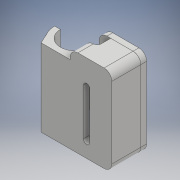
# Autodesk Inventor part: br
Saved by Autodesk Inventor 2018 (Build 220112000, 112)
## iProperties
Created: 2018-02-02
Part Number: br
Material: Generic
Document SubType Name: Modeling
Designer: eroldan
Density: 1 g/cm^3
Appearance: Default
Author: eroldan
Autodesk Inventor part; units mm, degrees
ref_plane "YZ Plane" through (0, 0, 0) normal (1, 0, 0) x (0, 1, 0)
ref_plane "XZ Plane" through (0, 0, 0) normal (0, 1, 0) x (-1, 0, 0)
sketch "Sketch4" plane through (0, 0, 0) normal (0, 0, 1) x (1, 0, 0)
  arc A0 (-8, 0) -> (8, 0) centre (0, 0) ccw
  line L0 (-11, 0) -> (-8, 0)
  line L1 (7.5498, -8) -> (25.5498, -8)
  line L2 (25.5498, -8) -> (25.5498, -11)
  arc A1 (-11, 0) -> (-9.5, -5.5453) centre (0, 0) ccw
  arc A2 (7.5498, -8) -> (11, 0) centre (0, 0) ccw
  line L3 (8, 0) -> (11, 0)
  line L4 (-7.0263, -11) -> (-9.5, -5.5453)
  line L5 (-7.0263, -11) -> (25.5498, -11)
  dimension "d0" = 16
  dimension "d14" = 18
  dimension "d15" = 3
  dimension "d20" = 3
  constraints: 12 end point, 6 point on circle, 4 horizontal, 3 centre point, 1 coincident, 1 perpendicular
  measures "d0" diameter of A0
  measures "d14" distance of L1.start L1.end
  measures "d15" distance of L1.end L2.end
  measures "d20" radial gap between concentric circles of A2 A0
extrude "Extrusion1" add sketch "Sketch4" along normal blind 40
sketch "Sketch5" plane through (7.5498, -8, 0) normal (0, 1, 0) x (1, 0, 0)
  line L0 (0, 0) -> (18, 0) projected
  line L1 (0, 0) -> (0, -40) projected
  line L2 (18, -40) -> (0, -40) projected
  line L3 (18, 0) -> (18, -40) projected
  line L4 (9, -32) -> (9, -8) construction
  line L5 (10.65, -32) -> (10.65, -8)
  line L6 (7.35, -8) -> (7.35, -32)
  arc A0 (7.35, -32) -> (10.65, -32) centre (9, -32) ccw
  arc A1 (10.65, -8) -> (7.35, -8) centre (9, -8) ccw
  point P0 (-7.5498, 0)
  point P1 (9, -20)
  point P2 (18, -20)
  dimension "d5" = 9
  dimension "d16" = 12
  dimension "d17" = 3.3
  constraints: 8 end point, 4 point on circle, 4 tangent, 2 centre point, 2 midpoint, 1 horizontal alignment, 1 parallel, 1 vertical
  measures "d5" distance of point (18, -20) point (9, -20)
  measures "d16" distance of point (9, -20) L4.end
  measures "d17" diameter of A1
extrude "Extrusion2" cut sketch "Sketch5" against normal through all contours A0 L6 A1 L5
ref_plane "Work Plane1" through (25.5498, -11, 8) normal (1, 0, 0) x (0, 0, -1)
sketch "Sketch7" plane through (25.5498, -11, 8) normal (1, 0, 0) x (0, 0, -1)
  line L0 (0, 3) -> (8, 3)
  line L1 (8, 11) -> (-7, 11)
  line L2 (-7, 11) -> (-7, 3)
  line L3 (-7, 3) -> (8, 3)
  line L4 (8, 3) -> (8, 11)
  dimension "d22" = 15
  constraints: 10 end point, 2 parallel, 1 horizontal, 1 perpendicular
  measures "d22" distance of L3.end L2.end
extrude "Extrusion3" cut sketch "Sketch7" against normal up to surface
sketch "Sketch8" plane through (-7.0263, -11, 0) normal (0, -1, 0) x (1, 0, 0)
  line L0 (32.5762, 0) -> (32.5762, 40) construction
  line L1 (32.5762, 40) -> (14.5762, 40) projected
  line L2 (36.5762, 0) -> (36.5762, 45)
  line L3 (36.5762, 45) -> (15.0263, 45)
  line L4 (36.5762, 0) -> (28.9847, 0)
  line L5 (28.9847, 0) -> (28.9847, 6)
  line L6 (28.9847, 6) -> (32.5762, 6)
  line L7 (32.5762, 6) -> (32.5762, 40)
  line L8 (15.0263, 15) -> (15.0263, 40) projected
  line L9 (15.0263, 40) -> (15.0263, 45)
  point P0 (7.0263, 0)
  dimension "d25" = 4
  dimension "d26" = 6
  dimension "d27" = 5
  constraints: 14 end point, 2 perpendicular, 1 collinear, 1 horizontal, 1 point on line, 1 vertical
  measures "d25" distance between parallel lines of L0 L2
  measures "d26" distance of L4.end L5.end
  measures "d27" distance between parallel lines of L3 L1
extrude "Extrusion4" add sketch "Sketch8" against normal blind 15
sketch "Sketch9" plane through (8, -11, 45) normal (0, 0, 1) x (1, 0, 0)
  line L0 (0, 15) -> (21.5498, 15) projected
  line L1 (0, 0) -> (0, 15) projected
  line L2 (0, 15) -> (6, 15)
  line L3 (6, 15) -> (6, 8)
  line L4 (6, 8) -> (0, 8)
  line L5 (0, 8) -> (0, 15)
  point P0 (-8, 11)
  dimension "d30" = 6
  dimension "d31" = 7
  constraints: 8 end point, 2 parallel, 1 horizontal, 1 perpendicular
  measures "d30" distance of L3.end L4.end
  measures "d31" distance of L2.end L3.end
extrude "Extrusion5" cut sketch "Sketch9" against normal up to surface (5 mm away)
fillet "Fillet2" radius 2 1 edges at (14, -3, 42.5)
fillet "Fillet3" radius 4 3 edges at (29.5498, -3.5, 45) (29.5498, -3.5, 0) (8, -7, 45)
sketch "Sketch10" plane through (-7.0263, 4, 0) normal (0, 1, 0) x (1, 0, 0)
  line L0 (28.9847, 0) -> (28.9847, -6) projected
  line L1 (21.0263, -40) -> (21.0263, -45) projected
  point P0 (7.0263, 0)
  point P1 (32.3891, -3.3174)
  point P2 (25.3561, -42.4627)
hole "Hole2" at (25.3628, 4, 3.3174) at (18.3298, 4, 42.4627) direction (0, -1, 0) diameter 3.1 depth 12 tip angle 118
sketch "Sketch11" plane through (-7.0263, 4, 0) normal (0, 1, 0) x (1, 0, 0)
  line L0 (36.5762, -41) -> (36.5762, -4) projected
  arc A0 (32.5762, -45) -> (36.5762, -41) centre (32.5762, -41) ccw projected
  line L1 (21.0263, -45) -> (32.5762, -45) projected
  arc A1 (36.5762, -4) -> (32.5762, 0) centre (32.5762, -4) ccw projected
  line L2 (32.5762, 0) -> (28.9847, 0) projected
  line L3 (15.0263, -15) -> (15.0263, -40) projected
  line L4 (15.0263, 0) -> (28.9847, 0)
  arc A2 (15.0263, -41) -> (19.0263, -45) centre (19.0263, -41) ccw projected
  line L5 (15.0263, -41) -> (15.0263, -40) projected
  line L6 (19.0263, -45) -> (21.0263, -45) projected
  line L7 (15.0263, 0) -> (15.0263, -15)
  circle A3 centre (32.3891, -3.3174) radius 1.55 projected
  circle A4 centre (25.3561, -42.4627) radius 1.55 projected
  point P0 (7.0263, 0)
  constraints: 4 end point, 1 point on line, 1 vertical
extrude "Extrusion6" add sketch "Sketch11" along normal blind 3 separate body
